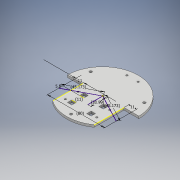
# Autodesk Inventor part: Base
Saved by Autodesk Inventor 2017 (Build 210142000, 142)
## iProperties
Part Number: Base
Material: Genérico
Document SubType Name: Modeling
Designer: fam
Density: 1 g/cm^3
Appearance: Valor por defecto
Author: fam
Autodesk Inventor part; units mm, degrees
ref_plane "YZ Plane" through (0, 0, 0) normal (1, 0, 0) x (0, 1, 0)
ref_plane "XZ Plane" through (0, 0, 0) normal (0, 1, 0) x (-1, 0, 0)
ref_plane "XY Plane" through (0, 0, 0) normal (0, 0, 1) x (1, 0, 0)
sketch "Boceto1" plane through (0, 0, 0) normal (0, 0, 1) x (1, 0, 0)
  circle A0 centre (0, 0) radius 50
  dimension "d0" = 100
  constraints: 1 centre point, 1 coincident
  measures "d0" diameter of A0
extrude "Extrusión1" add sketch "Boceto1" along normal blind 3.2
sketch "Boceto2" plane through (0, 0, 3.2) normal (0, 0, 1) x (1, 0, 0)
  circle A0 centre (-22, -11.99) radius 1.25
  circle A1 centre (-22, -29.99) radius 1.25
  circle A2 centre (22, -29.99) radius 1.25
  circle A3 centre (22, -11.99) radius 1.25
  line L0 (-29, 1.01) -> (-59, 1.01)
  line L1 (-59, 1.01) -> (-59, -41.99)
  line L2 (-59, -41.99) -> (-29, -41.99)
  line L3 (-29, -41.99) -> (-29, 1.01)
  line L4 (29, 1.01) -> (59, 1.01)
  line L5 (59, 1.01) -> (59, -41.99)
  line L6 (59, -41.99) -> (29, -41.99)
  line L7 (29, -41.99) -> (29, 1.01)
  circle A4 centre (0, 0) radius 4.16 construction
  line L8 (-4.16, 4.16) -> (4.16, 4.16) construction
  line L9 (4.16, 4.16) -> (4.16, -11.99) construction
  line L10 (4.16, -11.99) -> (-4.16, -11.99) construction
  line L11 (-4.16, -11.99) -> (-4.16, 4.16) construction
  dimension "d3" = 2.5
  dimension "d4" = 44
  dimension "d5" = 22
  dimension "d6" = 18
  dimension "d7" = 43
  dimension "d8" = 30
  dimension "d9" = 12
  dimension "d10" = 7
  dimension "d11" = 7
  dimension "d12" = 8.32
  dimension "d13" = 16.15
  constraints: 24 end point, 6 horizontal, 6 vertical, 5 centre point, 5 horizontal alignment, 3 equal radius, 3 tangent, 2 vertical alignment, 1 coincident, 1 collinear
  measures "d3" diameter of A3
  measures "d4" distance of A2.centre A1.centre
  measures "d5" horizontal distance of point (0, 0) A2.centre
  measures "d6" distance of A2.centre A3.centre
  measures "d7" distance of L4.end L5.end
  measures "d8" distance of L5.end L6.end
  measures "d9" distance from line of L6 A2.centre
  measures "d10" distance from line of L3 A1.centre
  measures "d11" distance from line of L7 A3.centre
  measures "d12" diameter of A4
  measures "d13" distance of L10.end L8.start
extrude "Extrusión2" cut sketch "Boceto2" against normal through all
sketch "Boceto3" plane through (0, 0, 3.2) normal (0, 0, 1) x (1, 0, 0)
  circle A0 centre (-7.83, 42) radius 1.25
  circle A1 centre (7.83, 42) radius 1.25
  arc A2 (49.9898, 1.01) -> (-49.9898, 1.01) centre (0, 0) ccw projected
  dimension "d16" = 15.66
  dimension "d17" = 2.5
  dimension "d18" = 7.83
  dimension "d19" = 42
  constraints: 2 centre point, 1 equal radius, 1 horizontal alignment
  measures "d16" distance of A1.centre A0.centre
  measures "d17" diameter of A1
  measures "d18" horizontal distance of point (0, 0) A0.centre
  measures "d19" vertical distance of A2.centre A0.centre
extrude "Extrusión3" cut sketch "Boceto3" against normal through all
sketch "Boceto4" plane through (0, 0, 3.2) normal (0, 0, 1) x (1, 0, 0)
  line L0 (-16.5, -9.49) -> (-10.5, -9.49)
  line L1 (-10.5, -9.49) -> (-10.5, -15.49)
  line L2 (-10.5, -15.49) -> (-16.5, -15.49)
  line L3 (-16.5, -15.49) -> (-16.5, -9.49)
  line L4 (10.5, -9.49) -> (16.5, -9.49)
  line L5 (16.5, -9.49) -> (16.5, -15.49)
  line L6 (16.5, -15.49) -> (10.5, -15.49)
  line L7 (10.5, -15.49) -> (10.5, -9.49)
  circle A0 centre (-22, -11.99) radius 1.25 projected
  circle A1 centre (22, -11.99) radius 1.25 projected
  line L8 (-16.5, -26.49) -> (-10.5, -26.49)
  line L9 (-10.5, -26.49) -> (-10.5, -32.49)
  line L10 (-10.5, -32.49) -> (-16.5, -32.49)
  line L11 (-16.5, -32.49) -> (-16.5, -26.49)
  line L12 (10.5, -26.49) -> (16.5, -26.49)
  line L13 (16.5, -26.49) -> (16.5, -32.49)
  line L14 (16.5, -32.49) -> (10.5, -32.49)
  line L15 (10.5, -32.49) -> (10.5, -26.49)
  circle A2 centre (-22, -29.99) radius 1.25 projected
  point P0 (0, 0)
  dimension "d22" = 6
  dimension "d23" = 5.5
  dimension "d24" = 5.5
  dimension "d25" = 2.5
  dimension "d26" = 6
  dimension "d27" = 6
  dimension "d28" = 6
  dimension "d32" = 2.5
  constraints: 32 end point, 8 horizontal, 8 vertical, 4 horizontal alignment, 2 collinear, 2 vertical alignment
  measures "d22" distance of L0.start L0.end
  measures "d23" distance from line of A0.centre L3
  measures "d24" distance from line of A1.centre L5
  measures "d25" distance from line of L0 A0.centre
  measures "d26" distance of L2.end L0.start
  measures "d27" distance of L8.start L8.end
  measures "d28" distance of L10.end L8.start
  measures "d32" distance from line of A2.centre L10
extrude "Extrusión4" cut sketch "Boceto4" against normal through all contours L0 L1 L2 L3 | L4 L5 L6 L7 | L8 L9 L10 L11 | L12 L13 L14 L15
sketch "Boceto5" plane through (0, 0, 3.2) normal (0, 0, 1) x (1, 0, 0)
  circle A0 centre (0, -44) radius 1.75
  arc A1 (49.9898, 1.01) -> (-49.9898, 1.01) centre (0, 0) ccw projected
  circle A2 centre (-37.5, 20.9519) radius 1.75
  circle A3 centre (37.5, 20.9519) radius 1.75
  point P0 (-27.1448, -41.99)
  point P1 (27.1448, -41.99)
  dimension "d33" = 3.5
  dimension "d34" = 44
  dimension "d35" = 37.5
  dimension "d36" = 37.5
  dimension "d37" = 75
  constraints: 3 centre point, 2 equal radius, 1 horizontal alignment, 1 vertical alignment
  measures "d33" diameter of A0
  measures "d34" distance of A1.centre A0.centre
  measures "d35" horizontal distance of point (0, 0) A2.centre
  measures "d36" horizontal distance of point (0, 0) A3.centre
  measures "d37" distance of A0.centre A3.centre
extrude "Extrusión5" cut sketch "Boceto5" against normal through all
sketch "Boceto6" plane through (0, 0, 3.2) normal (0, 0, 1) x (1, 0, 0)
  circle A0 centre (0, 0) radius 1
  dimension "d41" = 2
  constraints: 1 centre point, 1 coincident
  measures "d41" diameter of A0
extrude "Extrusión6" cut sketch "Boceto6" against normal through all
sketch "Boceto7" plane through (0, 0, 3.2) normal (0, 0, 1) x (1, 0, 0)
  circle A0 centre (0, 0) radius 1 projected
  line L0 (0, 0) -> (-40, -20.99)
  line L1 (-16.5, -26.49) -> (-10.5, -26.49) projected
  line L2 (-10.5, -15.49) -> (-16.5, -15.49) projected
  line L3 (-29, 1.01) -> (-29, -40.7308) projected
  line L4 (0, 0) -> (40, -20.99)
  line L5 (29, -40.7308) -> (29, 1.01) projected
  line L6 (0, 0) -> (0, -20.99)
  dimension "d44" = 11
  dimension "d45" = 5.5
  dimension "d46" = 11
  dimension "d47" = 45.1728
  dimension "d48" = 11
  dimension "d49" = 45.1728
  dimension "d50" = 80
  dimension "d51" = 20.99
  constraints: 6 end point, 2 horizontal alignment, 1 coincident, 1 vertical
  measures "d44" distance between parallel lines of L1 L2
  measures "d45" distance from line of L2 L0.end
  measures "d46" distance from line of L0.end L3
  measures "d47" distance of L0.start L0.end
  measures "d48" distance from line of L5 L4.end
  measures "d49" distance of L4.start L4.end
  measures "d50" distance of L4.end L0.end
  measures "d51" distance of L4.start L6.end
equation "\"d5\" = 0.5 * d4"
equation "\"d18\" = 0.5 * d16"
equation "\"d36\" = d35"
equation "\"d37\" = 2 * d35"
